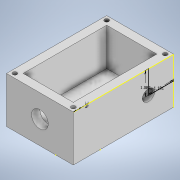
# Autodesk Inventor part: Water_Proof_Box_Bottom
Saved by Autodesk Inventor 2022 (Build 260153000, 153)
## iProperties
Created: 2023-07-12
Part Number: Water_Proof_Box_Bottom
Material: Generic
Document SubType Name: Modeling
Designer: jtw4137
Density: 1 g/cm^3
Appearance: Default
Author: jtw4137
Autodesk Inventor part; units mm, degrees
ref_plane "YZ Plane" through (0, 0, 0) normal (1, 0, 0) x (0, 1, 0)
ref_plane "XZ Plane" through (0, 0, 0) normal (0, 1, 0) x (-1, 0, 0)
ref_plane "XY Plane" through (0, 0, 0) normal (0, 0, 1) x (1, 0, 0)
sketch "Sketch1" plane through (0, 0, 0) normal (0, 1, 0) x (-1, 0, 0)
  line L0 (59.2038, 31.922) -> (59.2038, -88.078)
  line L1 (59.2038, -88.078) -> (-20.7962, -88.078)
  line L2 (-20.7962, -88.078) -> (-20.7962, 31.922)
  line L3 (-20.7962, 31.922) -> (59.2038, 31.922)
  point P0 (0, 0)
  dimension "d0" = 120
  dimension "d1" = 80
  constraints: 8 end point, 2 perpendicular, 1 vertical
  measures "d0" distance of L0.start L0.end
  measures "d1" distance of L2.end L0.start
extrude "Extrusion1" add sketch "Sketch1" along normal blind 55
shell "Shell2" thickness 10 removed faces 1 at (-5.8705, 55, -48.078)
sketch "Sketch12" plane through (0, 55, 0) normal (0, 1, 0) x (1, 0, 0)
  line L0 (10.7962, 78.078) -> (10.7962, -21.922) projected
  line L1 (10.7962, -21.922) -> (20.7962, -21.922)
  line L2 (20.7962, -31.922) -> (20.7962, 88.078) projected
  line L3 (20.7962, -21.922) -> (20.7962, -31.922)
  line L4 (20.7962, -31.922) -> (10.7962, -31.922)
  line L5 (10.7962, -31.922) -> (10.7962, -21.922)
  line L6 (20.7962, -31.922) -> (15.8432, -31.922)
  line L7 (-59.2038, -31.922) -> (20.7962, -31.922) projected
  line L8 (15.8432, -26.969) -> (20.7962, -26.969)
  line L9 (15.8432, -26.969) -> (15.8432, -31.922)
  point P0 (0, 0)
  dimension "d124" = 4.953
  dimension "d125" = 4.953
  constraints: 14 end point, 5 perpendicular, 2 point on line, 1 horizontal
  measures "d124" distance of L8.start L6.end
  measures "d125" distance of L8.start L8.end
hole "Hole11" at (15.8432, 55, 26.969) direction (0, -1, 0) diameter 5 end through all
sketch "Sketch19" plane through (0, 55, 0) normal (0, 1, 0) x (1, 0, 0)
  line L0 (10.7962, -21.922) -> (-49.2038, -21.922) projected
  line L1 (-49.2038, -21.922) -> (-49.2038, -31.922)
  line L2 (-59.2038, -31.922) -> (20.7962, -31.922) projected
  line L3 (-59.2038, -31.922) -> (-59.2038, -21.922)
  line L4 (-59.2038, 88.078) -> (-59.2038, -31.922) projected
  line L5 (-49.2038, -23.8125) -> (-49.2038, -21.922)
  line L6 (-59.2038, -21.922) -> (-49.2038, -21.922)
  line L7 (-49.2038, -21.922) -> (-49.2038, 78.078) projected
  line L8 (-49.2038, -21.922) -> (-54.2038, -21.922)
  line L9 (-54.1566, -26.875) -> (-49.2038, -26.922)
  line L10 (-54.1566, -26.875) -> (-54.2038, -21.922)
  point P0 (0, 0)
  dimension "d133" = 4.953
  dimension "d134" = 4.953
  constraints: 14 end point, 3 point on line, 2 midpoint, 1 parallel, 1 perpendicular, 1 vertical
  measures "d133" distance of L9.start L9.end
  measures "d134" vertical distance of L9.start L8.end
hole "Hole12" at (-54.1566, 55, 26.875) direction (0, -1, 0) diameter 5 end through all
sketch "Sketch21" plane through (0, 55, 0) normal (0, 1, 0) x (1, 0, 0)
  line L0 (10.7962, -21.922) -> (10.7962, 78.078) projected
  line L1 (10.7962, 78.078) -> (20.7962, 78.078)
  line L2 (20.7962, -31.922) -> (20.7962, 88.078) projected
  line L3 (20.7962, 88.078) -> (10.7962, 88.078)
  line L4 (20.7962, 88.078) -> (-59.2038, 88.078) projected
  line L5 (10.7962, 78.078) -> (10.7962, 88.078)
  line L6 (10.7962, 78.078) -> (-49.2038, 78.078) projected
  line L7 (10.7962, 78.078) -> (15.7962, 78.078)
  line L8 (15.8432, 83.031) -> (20.7962, 83.031)
  line L9 (15.8432, 83.031) -> (15.7962, 78.078)
  point P0 (0, 0)
  dimension "d146" = 4.953
  constraints: 12 end point, 3 point on line, 2 perpendicular, 1 horizontal, 1 midpoint
  measures "d146" distance of L8.start L8.end
hole "Hole13" at (15.8432, 55, -83.031) direction (0, -1, 0) diameter 5 end through all
sketch "Sketch22" plane through (0, 55, 0) normal (0, 1, 0) x (1, 0, 0)
  line L0 (-49.2038, 78.078) -> (10.7962, 78.078) projected
  line L1 (-49.2038, 78.078) -> (-59.2038, 78.078)
  line L2 (-59.2038, 88.078) -> (-59.2038, -31.922) projected
  line L3 (-59.2038, 88.078) -> (-49.2038, 88.078)
  line L4 (20.7962, 88.078) -> (-59.2038, 88.078) projected
  line L5 (-49.2038, 78.078) -> (-49.2038, 88.078)
  line L6 (-49.2038, 78.078) -> (-54.2038, 78.078)
  line L7 (-54.1568, 83.031) -> (-49.2038, 83.031)
  line L8 (-54.1568, 83.031) -> (-54.2038, 78.078)
  point P0 (0, 0)
  dimension "d155" = 4.953
  dimension "d156" = 4.953
  constraints: 12 end point, 3 point on line, 2 perpendicular, 1 horizontal, 1 midpoint
  measures "d155" distance of L7.start L7.end
  measures "d156" vertical distance of L7.start L6.end
hole "Hole14" at (-54.1568, 55, -83.031) direction (0, -1, 0) diameter 5 end through all
sketch "Sketch23" plane through (-59.2038, 0, 31.922) normal (0, 0, 1) x (1, 0, 0)
  point P0 (59.2038, 0)
sketch "Sketch24" plane through (-59.2038, 0, 31.922) normal (0, 0, 1) x (1, 0, 0)
  line L0 (0, 0) -> (0, 55) projected
  line L1 (0, 55) -> (0, 0)
  line L2 (0, 0) -> (80, 0) projected
  line L3 (0, 0) -> (80, 0)
  line L4 (80, 0) -> (80, 55) projected
  line L5 (80, 0) -> (80, 55)
  line L6 (0, 55) -> (80, 55) projected
  line L7 (80, 55) -> (0, 55)
  line L8 (0, 27.5045) -> (39.9999, 27.5045)
  line L9 (39.9999, 27.5045) -> (40, 55)
  line L10 (70, 55) -> (10, 55) projected
  point P0 (59.2038, 0)
  dimension "d164" = 54.991
  dimension "d165" = 80
  dimension "d175" = 39.9999
  dimension "d176" = 27.4955
  constraints: 12 end point, 3 collinear, 2 perpendicular, 1 midpoint, 1 point on line
  measures "d165" distance of L0.end L4.end
  measures "d175" distance of L8.start L8.end
  measures "d176" distance of L8.end L9.end
hole "Hole15" at (-19.2039, 27.5045, 31.922) direction (0, 0, -1) diameter 20 depth 25.4 tip angle 118
sketch "Sketch32" plane through (20.7962, 0, 31.922) normal (1, 0, 0) x (0, 0, -1)
  line L0 (0, 55) -> (120, 55) projected
  line L1 (90, 55) -> (90, 27.5)
  line L2 (90, 27.5) -> (120, 27.5)
  line L3 (120, 0) -> (120, 55) projected
  point P0 (31.922, 0)
  dimension "d189" = 27.5
  dimension "d190" = 30
  constraints: 4 end point, 2 perpendicular, 1 midpoint, 1 point on line
  measures "d189" distance of L1.start L1.end
  measures "d190" distance of L1.end L2.end
sketch "Sketch33" plane through (20.7962, 0, 31.922) normal (1, 0, 0) x (0, 0, -1)
  line L0 (89.9856, 20.7094) -> (89.9856, 34.3094) construction
  line L1 (82.4856, 28.2094) -> (82.4856, 26.8094)
  line L2 (97.4856, 26.8094) -> (97.4856, 28.2094)
  arc A0 (82.4856, 28.2094) -> (97.4856, 28.2094) centre (89.9856, 28.2094) ccw
  arc A1 (97.4856, 26.8094) -> (82.4856, 26.8094) centre (89.9856, 26.8094) ccw
  point P0 (31.922, 0)
  point P1 (89.9856, 27.5094)
  point P2 (97.4528, 27.5094)
  point P3 (82.5183, 27.5094)
  dimension "d191" = 13.6
  dimension "d192" = 7.5
  constraints: 8 end point, 6 point on circle, 4 tangent, 2 centre point, 2 point on line, 1 midpoint, 1 parallel, 1 vertical
  measures "d191" distance of L0.start L0.end
  measures "d192" distance from line of L2 point (89.986, 27.509)
extrude "Extrusion2" cut sketch "Sketch33" against normal blind 10 contours A1 A0
body "Solid1"
